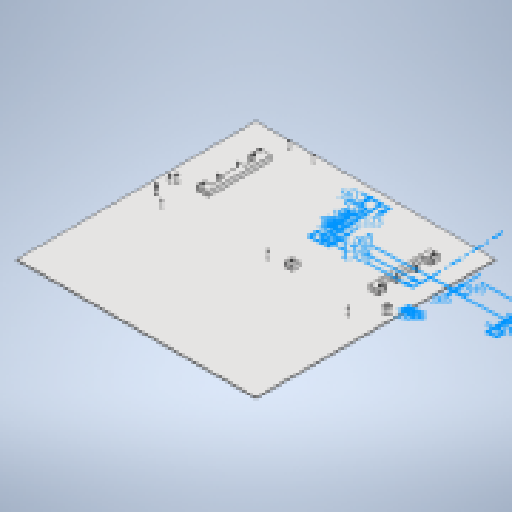
# Autodesk Inventor part: chassis
Saved by Autodesk Inventor 2025 (Build 290162010, 162A)
## iProperties
Created: 2025-12-11
Part Number: chassis
Material: Generic
Document SubType Name: Modeling
Designer: 200481997
Density: 1 g/cm^3
Appearance: Default
Author: 200481997
Autodesk Inventor part; units mm, degrees
ref_plane "YZ Plane" through (0, 0, 0) normal (1, 0, 0) x (0, 1, 0)
ref_plane "XZ Plane" through (0, 0, 0) normal (0, 1, 0) x (-1, 0, 0)
ref_plane "XY Plane" through (0, 0, 0) normal (0, 0, 1) x (1, 0, 0)
sketch "Sketch3" plane through (0, 0, 0) normal (0, 1, 0) x (-1, 0, 0)
  line L0 (-140, -85.7143) -> (160, -85.7143)
  line L1 (160, -85.7143) -> (160, 214.2857)
  line L2 (160, 214.2857) -> (-140, 214.2857)
  line L3 (-140, 214.2857) -> (-140, -85.7143)
  point P0 (0, 0)
  dimension "d80" = 300
  dimension "d81" = 300
  dimension "d82" = 140
  dimension "d83" = 85.7143
  constraints: 8 end point, 2 parallel, 1 horizontal, 1 perpendicular
  measures "d80" distance between parallel lines of L2 L0
  measures "d81" distance between parallel lines of L1 L3
  measures "d82" distance from line of point (0, 0) L3
  measures "d83" distance from line of point (0, 0) L0
extrude "Chassis base" add sketch "Sketch3" against normal blind 1.5875
sketch "Motherboard Mounting Holes" plane through (0, 0, 0) normal (0, 1, 0) x (-1, 0, 0)
  circle A0 centre (142.65, 56.4682) radius 1.15
  circle A1 centre (142.65, 56.4682) radius 2.5
  circle A2 centre (118.8, -41.6318) radius 2.05
  circle A3 centre (143.65, 30.0682) radius 1.15
  circle A4 centre (142.65, 56.4682) radius 2.5
  circle A5 centre (118.8, -41.6318) radius 0.7
  circle A6 centre (143.65, 30.0682) radius 2.5
  circle A7 centre (148.65, 51.0682) radius 1.1
  circle A8 centre (118.8, 22.3682) radius 0.7
  circle A9 centre (118.8, -41.6318) radius 2.05
  circle A10 centre (148.65, 34.0682) radius 1.1
  circle A11 centre (119.95, -50.0818) radius 1.25
  circle A12 centre (-102.85, -46.4318) radius 2
  circle A13 centre (-102.85, -46.4318) radius 0.9
  circle A14 centre (-103.35, 21.2682) radius 1.85
  circle A15 centre (-131, 40.4962) radius 4
  circle A16 centre (-103.35, 21.2682) radius 0.9
  circle A17 centre (-131, 40.4962) radius 1.35
  circle A18 centre (-103.35, -41.5818) radius 1.25
  circle A19 centre (-20.85, 50.0682) radius 0.9
  circle A20 centre (118.8, 22.3682) radius 2.05
  circle A21 centre (-20.85, 50.0682) radius 2
  circle A22 centre (118.8, -41.6318) radius 2.05
  circle A23 centre (142.65, 56.4682) radius 2.5
  circle A24 centre (118.8, -41.6318) radius 2.05
  circle A25 centre (148.65, 51.0682) radius 1.8
  circle A26 centre (148.65, 34.0682) radius 1.8
  line L0 (119.55, -51.2661) -> (119.55, -48.8975)
  line L1 (120.35, -48.8975) -> (120.35, -51.2661)
  line L2 (120.35, -51.6947) -> (119.55, -48.4689) construction
  line L3 (119.55, -51.6947) -> (120.35, -48.4689) construction
  line L4 (121.1343, -49.6818) -> (118.7657, -49.6818)
  line L5 (118.7657, -50.4818) -> (121.1343, -50.4818)
  line L6 (122.1914, -49.6818) -> (117.7086, -50.4818) construction
  line L7 (117.7086, -49.6818) -> (122.1914, -50.4818) construction
  line L8 (-103.75, -42.7661) -> (-103.75, -40.3975)
  line L9 (-102.95, -40.3975) -> (-102.95, -42.7661)
  line L10 (-102.95, -43.2946) -> (-103.75, -39.869) construction
  line L11 (-103.75, -43.2946) -> (-102.95, -39.869) construction
  line L12 (-102.1657, -41.1818) -> (-104.5343, -41.1818)
  line L13 (-104.5343, -41.9818) -> (-102.1657, -41.9818)
  line L14 (-101.5, -41.1818) -> (-105.2, -41.9818) construction
  line L15 (-105.2, -41.1818) -> (-101.5, -41.9818) construction
  point P0 (0, 0)
  point P1 (-102.95, -41.1818)
  point P2 (-103.75, -41.1818)
  point P3 (-103.75, -41.9818)
  point P4 (-102.95, -41.9818)
  point P5 (119.55, -50.4818)
  point P6 (120.35, -50.4818)
  point P7 (120.35, -49.6818)
  point P8 (119.55, -49.6818)
  dimension "d12" = 2.5
  dimension "d39" = 2.5
  dimension "d0" = 41.6318
  dimension "d1" = 118.8
  dimension "d2" = 8.45
  dimension "d3" = 1.15
  dimension "d8" = 102.85
  dimension "d9" = 46.4318
  dimension "d10" = 1.8
  dimension "d11" = 4
  dimension "d13" = 4.85
  dimension "d14" = 0.5
  dimension "d15" = 50.0682
  dimension "d16" = 20.85
  dimension "d17" = 1.8
  dimension "d18" = 4
  dimension "d19" = 103.35
  dimension "d20" = 21.2682
  dimension "d21" = 1.8
  dimension "d22" = 3.7
  dimension "d23" = 118.8
  dimension "d24" = 22.3682
  dimension "d25" = 1.4
  dimension "d26" = 4.1
  dimension "d27" = 143.65
  dimension "d28" = 30.0682
  dimension "d29" = 2.3
  dimension "d30" = 5
  dimension "d31" = 4
  dimension "d32" = 5
  dimension "d33" = 2.2
  dimension "d34" = 3.6
  dimension "d35" = 17
  dimension "d36" = 5.4
  dimension "d37" = 1.4
  dimension "d38" = 4.1
  dimension "d40" = 131
  dimension "d41" = 40.4962
  dimension "d42" = 6
  dimension "d52" = 8
  dimension "d53" = 2.7
  dimension "d66" = 0.8
  dimension "d67" = 0.8
  dimension "d68" = 0.8
  dimension "d69" = 0.8
  dimension "d71" = 0.4
  dimension "d72" = 0.4
  dimension "d73" = 0.4
  dimension "d74" = 0.4
  constraints: 32 end point, 25 centre point, 10 concentric, 8 midpoint, 4 equal radius, 4 parallel, 2 horizontal, 1 vertical alignment, 20 other
  measures "d0" vertical distance of point (0, 0) A2.centre
  measures "d1" horizontal distance of point (0, 0) A2.centre
  measures "d2" vertical distance of A2.centre point (119.95, -50.082)
  measures "d3" horizontal distance of point (119.95, -50.082) A2.centre
  measures "d8" horizontal distance of point (0, 0) A12.centre
  measures "d9" vertical distance of point (0, 0) A12.centre
  measures "d10" diameter of A13
  measures "d11" diameter of A12
  measures "d13" vertical distance of point (-103.35, -41.582) A12.centre
  measures "d14" horizontal distance of A12.centre point (-103.35, -41.582)
  measures "d15" vertical distance of point (0, 0) A19.centre
  measures "d16" horizontal distance of point (0, 0) A19.centre
  measures "d17" diameter of A19
  measures "d18" diameter of A21
  measures "d19" horizontal distance of point (0, 0) A14.centre
  measures "d20" vertical distance of A14.centre point (0, 0)
  measures "d21" diameter of A16
  measures "d22" diameter of A14
  measures "d23" horizontal distance of point (0, 0) A8.centre
  measures "d24" vertical distance of point (0, 0) A8.centre
  measures "d25" diameter of A8
  measures "d26" diameter of A20
  measures "d27" horizontal distance of point (0, 0) A3.centre
  measures "d28" vertical distance of point (0, 0) A3.centre
  measures "d29" diameter of A3
  measures "d30" diameter of A6
  measures "d31" vertical distance of A3.centre A10.centre
  measures "d32" horizontal distance of A3.centre A10.centre
  measures "d33" diameter of A10
  measures "d34" diameter of A26
  measures "d35" distance of A7.centre A26.centre
  measures "d36" vertical distance of A7.centre A0.centre
  measures "d37" diameter of A5
  measures "d38" diameter of A2
  measures "d40" horizontal distance of point (0, 0) A15.centre
  measures "d41" vertical distance of point (0, 0) A15.centre
  measures "d42" horizontal distance of A7.centre A0.centre
  measures "d52" diameter of A15
  measures "d53" diameter of A17
  measures "d66" distance between parallel lines of L4 L5
  measures "d67" distance between parallel lines of L0 L1
  measures "d68" distance between parallel lines of L12 L13
  measures "d69" distance between parallel lines of L8 L9
  measures "d71" distance from line of point (-103.35, -41.582) L12
  measures "d72" distance from line of point (-103.35, -41.582) L9
  measures "d73" distance from line of point (119.95, -50.082) L5
  measures "d74" distance from line of L0 point (119.95, -50.082)
sketch "DP adapter Mounting Holes" plane through (0, 0, 0) normal (0, 1, 0) x (1, 0, 0)
  circle A0 centre (-109.8518, 77.3373) radius 1.27
  circle A1 centre (-79.6718, 77.3373) radius 1.27
  circle A2 centre (-109.8518, 77.3373) radius 0.7
  circle A3 centre (-79.6718, 77.3373) radius 0.7
  point P0 (0, 0)
  dimension "d45" = 2.54
  dimension "d46" = 30.18
  dimension "d47" = 1.4
  constraints: 4 centre point, 2 coincident, 2 equal radius, 1 horizontal alignment
  measures "d45" diameter of A0
  measures "d46" distance of A0.centre A1.centre
  measures "d47" diameter of A2
sketch "Battery Mounting" plane through (0, 0, 0) normal (0, 1, 0) x (1, 0, 0)
  circle A0 centre (-125.44, -67.1299) radius 0.8509
  circle A1 centre (-125.44, -67.1299) radius 1.27
  circle A2 centre (-3.4438, -55.8523) radius 1.27
  circle A3 centre (-3.4438, -55.8523) radius 0.8509
  circle A4 centre (108.5448, -67.1299) radius 0.8509
  circle A5 centre (108.5448, -67.1299) radius 1.27
  point P0 (0, 0)
  dimension "d86" = 1.7018
  dimension "d87" = 2.54
  dimension "d88" = 121.9962
  dimension "d89" = 11.2776
  dimension "d90" = 111.9886
  dimension "d91" = 11.2776
  dimension "d92" = 55.8523
  dimension "d93" = 3.4438
  constraints: 6 centre point, 4 equal radius, 3 coincident
  measures "d86" diameter of A0
  measures "d87" diameter of A1
  measures "d88" horizontal distance of A0.centre A2.centre
  measures "d89" vertical distance of A0.centre A2.centre
  measures "d90" horizontal distance of A2.centre A4.centre
  measures "d91" vertical distance of A2.centre A4.centre
  measures "d92" vertical distance of point (0, 0) A2.centre
  measures "d93" horizontal distance of A2.centre point (0, 0)
extrude "Motherboard Mounting Extrusions" add sketch "Motherboard Mounting Holes" along normal blind 7.1 contours A2 | A12 | A14 | A20 | A21
extrude "Motherboard Support Extrusions" add sketch "Motherboard Mounting Holes" along normal blind 7.75 contours A11 L5 L1 L4 | L1 L4 L0 A11 | L1 L5 L0 L4 | A11 L0 L5 L1 | L0 L5 A11 L4 | A18 L13 L9 L12 | L9 L12 L8 A18 | L9 L13 L8 L12 | A18 L8 L13 L9 | L8 L13 A18 L12
chamfer "Motherboard Support Chamfer" distance 0.3556 angle 45 8 edges at (103.35, 7.75, -42.8318) (104.6, 7.75, -41.5818) (103.35, 7.75, -40.3318) (102.1, 7.75, -41.5818) (-118.7, 7.75, -50.0818) (-119.95, 7.75, -51.3318) (-121.2, 7.75, -50.0818) (-119.95, 7.75, -48.8318)
extrude "Headphone Mounting Extrusions" add sketch "Motherboard Mounting Holes" along normal blind 7.9 contours A1 | A6
extrude "Headphone Support Base" add sketch "Motherboard Mounting Holes" along normal blind 5.4 contours A7 | A10 | A25 | A26
extrude "Headphone Support" add sketch "Motherboard Mounting Holes" along normal blind 2.1 from surface at 5.4 contours A7 | A10
fillet "Round Headphone Support" radius 0.381 2 edges at (-147.55, 7.5, 34.0682) (-147.55, 7.5, 51.0682)
extrude "Wifi Card Mounting Extrusion" add sketch "Motherboard Mounting Holes" along normal blind 8.685 contours A15
chamfer "Wifi Card Mount Chamfer" distance 1.143 angle 45 1 edges at (135, 8.685, 40.4962)
extrude "DP adapter Mouting Extrusions" add sketch "DP adapter Mounting Holes" along normal blind 7.62
extrude "Battery Mounting Extrusions" add sketch "Battery Mounting" along normal blind 8.382
sketch "Motherboard Screw Support" plane through (0, 0, 0) normal (0, 1, 0) x (1, 0, 0)
  arc A0 (-121.95, 52.4118) -> (-122.45, 51.9118) centre (-121.95, 51.9118) ccw
  line L0 (-122.45, 48.7118) -> (-122.45, 51.9118)
  line L1 (-121.55, 44.3318) -> (-121.55, 47.7168)
  arc A1 (-121.55, 47.7168) -> (-122, 48.2143) centre (-122.05, 47.7168) ccw
  arc A2 (-122.45, 48.7118) -> (-122, 48.2143) centre (-121.95, 48.7118) ccw
  arc A3 (-121.1, 22.9318) -> (-120.6, 22.4318) centre (-120.6, 22.9318) ccw
  line L2 (-120.6, 22.4318) -> (-120.05, 22.4318)
  line L3 (-116.05, 11.6368) -> (-116.05, 2.9818)
  line L4 (-121.55, -26.9182) -> (-121.55, -25.0682)
  line L5 (-121.1, -19.6682) -> (-121.1, -25.0682)
  line L6 (-121.1, -25.0682) -> (-121.55, -25.0682)
  arc A4 (-120.784, -0.6538) -> (-121.1, -1.0041) centre (-120.5966, -1.1406) ccw
  line L7 (-121.1, -1.1682) -> (-121.1, -1.0041)
  arc A5 (-116.05, 17.8982) -> (-120.05, 22.4318) centre (-120.6192, 17.8982) ccw
  line L8 (-116.05, 17.8982) -> (-116.05, 11.6368)
  line L9 (-121.1, 38.9318) -> (-121.55, 44.3318)
  line L10 (-121.1, -17.1557) -> (-112.4692, -17.1557)
  line L11 (-112.4692, -17.1557) -> (-112.4692, -2.3695)
  line L12 (-112.4692, -2.3695) -> (-121.1, -2.3695)
  line L13 (-121.1, -19.6682) -> (-121.1, -17.1557)
  line L14 (-121.1, -2.3695) -> (-121.1, -1.1682)
  line L15 (-121.55, -26.9182) -> (-107.4531, -26.9182)
  line L16 (-107.4531, -26.9182) -> (-107.4531, 52.4118)
  line L17 (-107.4531, 52.4118) -> (-121.95, 52.4118)
  arc A6 (-120.4125, -0.6538) -> (-116.05, 2.9818) centre (-120.622, 4.0327) ccw
  line L18 (-120.4125, -0.6538) -> (-120.784, -0.6538)
  line L19 (-121.1, 23.9922) -> (-112.4692, 23.9922)
  line L20 (-121.1, 23.9922) -> (-121.1, 22.9318)
  line L21 (-112.4692, 38.1735) -> (-121.1, 38.1735)
  line L22 (-121.1, 38.1735) -> (-121.1, 38.9318)
  line L23 (-112.4692, 23.9922) -> (-112.4692, 38.1735)
  line L24 (0, 0) -> (0, 98.7957)
  line L25 (101.95, 49.6818) -> (105.75, 49.6818)
  line L26 (106.25, 49.1818) -> (106.25, 42.6793)
  line L27 (99.85, 3.5318) -> (99.85, 9.0318)
  line L28 (106.25, -23.9682) -> (106.25, -26.9182)
  line L29 (106.25, -23.9682) -> (105.8, -18.5682)
  line L30 (105.8, -16.9179) -> (97.2157, -16.9179)
  line L31 (97.2157, -16.9179) -> (97.2157, -2.1645)
  line L32 (97.2157, -2.1645) -> (105.8, -2.1645)
  arc A7 (105.8, -1.2682) -> (105.0841, -0.7299) centre (105.0841, -1.4752) ccw
  line L33 (105.0841, -0.7299) -> (103.5506, -0.7299)
  arc A8 (99.85, 3.5318) -> (103.5506, -0.7299) centre (103.9522, 3.3563) ccw
  arc A9 (105.2607, 22.3458) -> (105.8, 22.8318) centre (105.2406, 22.9103) ccw
  line L34 (105.2607, 22.3458) -> (103.5965, 22.3458)
  arc A10 (103.5965, 22.3458) -> (99.85, 19.4482) centre (103.5593, 18.523) ccw
  line L35 (99.85, 9.0318) -> (99.85, 19.4482)
  line L36 (105.8, 24.1037) -> (97.4099, 24.1037)
  line L37 (97.4099, 24.1037) -> (97.4099, 38.0999)
  line L38 (97.4099, 38.0999) -> (105.8, 38.0999)
  line L39 (105.8, 41.8441) -> (106.25, 42.6793)
  arc A11 (106.25, 49.1818) -> (105.75, 49.6818) centre (105.75, 49.1818) ccw
  line L40 (101.95, 49.6818) -> (98.7893, 49.6818)
  line L41 (98.7893, 49.6818) -> (94.5011, 49.6818)
  line L42 (94.5011, 49.6818) -> (94.5011, -26.9182)
  line L43 (94.5011, -26.9182) -> (106.25, -26.9182)
  line L44 (105.8, -18.5682) -> (105.8, -16.9179)
  line L45 (105.8, -2.1645) -> (105.8, -1.2682)
  line L46 (105.8, 22.8318) -> (105.8, 24.1037)
  line L47 (105.8, 38.0999) -> (105.8, 41.8441)
  line L48 (16.278, -45.4962) -> (25.422, -45.4962)
  line L49 (25.422, -45.4962) -> (25.422, -54.6402)
  line L50 (25.422, -54.6402) -> (16.278, -54.6402)
  line L51 (16.278, -54.6402) -> (16.278, -45.4962)
  circle A12 centre (20.85, -50.0682) radius 0.9 projected
  dimension "d96" = 79.33
  dimension "d97" = 107.4531
  dimension "d98" = 112.4692
  dimension "d99" = 14.7862
  dimension "d100" = 2.3695
  dimension "d103" = 4.5692
  dimension "d104" = 4.5692
  dimension "d105" = 4.5466
  dimension "d107" = 4.572
  dimension "d108" = 4.6912
  dimension "d109" = 1.7157
  dimension "d110" = 1.229
  dimension "d111" = 0.5216
  dimension "d112" = 8.6308
  dimension "d113" = 14.1813
  dimension "d114" = 14.2383
  dimension "d115" = 5.3489
  dimension "d116" = 2.7146
  dimension "d117" = 14.7534
  dimension "d118" = 2.1645
  dimension "d119" = 1.4345
  dimension "d120" = 0.7452
  dimension "d121" = 0.6893
  dimension "d122" = 5.5208
  dimension "d123" = 4.106
  dimension "d124" = 13.9962
  dimension "d125" = 2.9089
  dimension "d126" = 3.8229
  dimension "d127" = 3.7093
  dimension "d128" = 1.7579
  dimension "d129" = 24.1037
  dimension "d130" = 1.1934
  dimension "d131" = 0.5649
  dimension "d132" = 5.5807
  dimension "d135" = 4.572
  dimension "d136" = 4.572
  dimension "d137" = 9.144
  dimension "d138" = 9.144
  constraints: 104 end point, 24 point on circle, 19 vertical, 14 horizontal, 12 centre point, 7 perpendicular, 2 collinear, 2 parallel, 2 tangent, 1 point on line, 36 other
  measures "d96" distance of L15.end L16.end
  measures "d97" distance from line of L24.start L16
  measures "d98" distance from line of L24.start L11
  measures "d99" distance between parallel lines of L10 L12
  measures "d100" distance from line of L24.start L12
  measures "d103" radius of A5
  measures "d104" distance from line of L8 A5.centre
  measures "d105" distance from line of L3 A4.centre
  measures "d107" distance from line of L3 A6.centre
  measures "d108" radius of A6
  measures "d109" distance between parallel lines of L12 L18
  measures "d110" distance from line of L12 A4.centre
  measures "d111" radius of A4
  measures "d112" distance of L19.start L19.end
  measures "d113" distance between parallel lines of L21 L19
  measures "d114" distance between parallel lines of L17 L21
  measures "d115" distance between parallel lines of L42 L35
  measures "d116" distance between parallel lines of L42 L31
  measures "d117" distance between parallel lines of L30 L32
  measures "d118" distance from line of L24.start L32
  measures "d119" distance between parallel lines of L32 L33
  measures "d120" radius of A7
  measures "d121" distance from line of L32 A7.centre
  measures "d122" distance from line of L32 A8.centre
  measures "d123" radius of A8
  measures "d124" distance between parallel lines of L36 L38
  measures "d125" distance between parallel lines of L42 L37
  measures "d126" radius of A10
  measures "d127" distance from line of A10.centre L35
  measures "d128" distance between parallel lines of L34 L36
  measures "d129" distance from line of L24.start L36
  measures "d130" distance from line of L36 A9.centre
  measures "d131" radius of A9
  measures "d132" distance from line of L36 A10.centre
  measures "d135" distance from line of A12.centre L49
  measures "d136" distance from line of L50 A12.centre
  measures "d137" distance between parallel lines of L50 L48
  measures "d138" distance between parallel lines of L49 L51
ref_plane "Work Plane1" through (-129.1327, 6.1, -60.3097) normal (0, -1, 0) x (1, 0, 0)
extrude "Motherboard Screw Support Extrusions" add sketch "Motherboard Screw Support" along normal up to surface (6.1 mm away)
body "Solid1"
